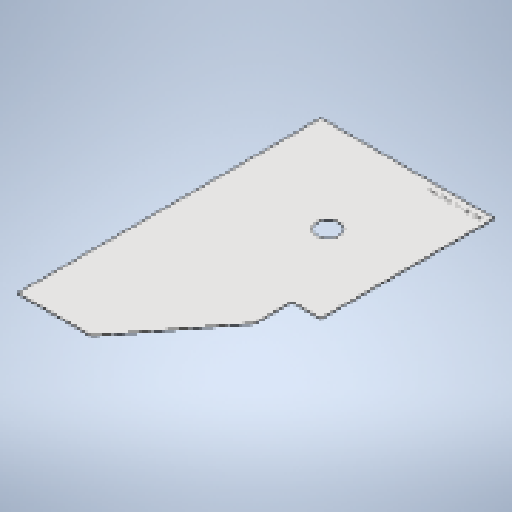
# Autodesk Inventor part: TRM 015 left board main
Saved by Autodesk Inventor 2025 (Build 290162010, 162A)
## iProperties
Created: 2024-08-07
Part Number: TRM 015 left board main
Material: AISI 304
Document SubType Name: Sheet Metal
Designer: pokla
Density: 8.02768 g/cm^3
Flat Pattern Width: 60.129 cm
Flat Pattern Length: 105 cm
Flat Pattern Area: 6313.54 cm^2
Sheet Metal Rule: AISI304 2mm Die16
Sheet Metal Width: 601,290 mm
Sheet Metal Length: 1050,000 mm
Sheet Metal Area: 631354,486 mm^2
Appearance: Default
Stock Number: ТРМ 015 левый борт основное
Author: pokla
Autodesk Inventor part; units mm, degrees
ref_plane "YZ Plane" through (0, 0, 0) normal (1, 0, 0) x (0, 1, 0)
ref_plane "XZ Plane" through (0, 0, 0) normal (0, 1, 0) x (-1, 0, 0)
ref_plane "XY Plane" through (0, 0, 0) normal (0, 0, 1) x (1, 0, 0)
sketch "Sketch1" plane through (0, 0, 0) normal (0, 0, 1) x (1, 0, 0)
  line L0 (-344.9768, -443.1916) -> (256.3132, -443.1916)
  line L1 (256.3132, -443.1916) -> (256.3132, 606.8084)
  line L2 (256.3132, 606.8084) -> (-344.9768, 606.8084)
  line L3 (-344.9768, 606.8084) -> (-344.9768, -443.1916)
  line L4 (-90.4868, -443.1916) -> (256.3132, 5.4517)
  circle A0 centre (0, 286.8084) radius 40
  line L5 (256.3132, 5.4517) -> (156.3132, 5.4517)
  line L6 (156.3132, 5.4517) -> (156.3132, -123.9149)
  point P0 (0, 0)
  dimension "d1" = 1050
  dimension "d14" = 80
  dimension "d15" = 320
  dimension "d16" = 100
  measures "d1" distance of L1.end L0.end
  measures "d14" diameter of A0
  measures "d15" distance from line of A0.centre L2
  measures "d16" distance of L4.end L5.end
extrude "Plate1" add sketch "Sketch1" along normal blind 2 contours L3 L2 L1 L5 L6 L4 L0
sketch "Sketch2" plane through (0, 0, 0) normal (0, 0, -1) x (-1, 0, 0)
  line L0 (-236.3132, 586.8084) -> (-36.3132, 586.8084) construction
  line L1 (-36.3132, 586.8084) -> (-36.3132, 566.8084) construction
  line L2 (-36.3132, 566.8084) -> (-236.3132, 566.8084) construction
  line L3 (-236.3132, 566.8084) -> (-236.3132, 586.8084) construction
  line L4 (-256.3132, 606.8084) -> (344.9768, 606.8084) projected
  line L5 (-256.3132, 5.4517) -> (-256.3132, 606.8084) projected
  point P0 (0, 0)
  point P1 (-48, 100)
  point P2 (-251, -525)
  point P3 (-50, 98)
  dimension "d6" = 200
  dimension "d9" = 20
  dimension "d10" = 20
  dimension "d11" = 20
  constraints: 4 other
  measures "d6" distance of L0.start L0.end
  measures "d9" distance of L0.end L1.end
  measures "d11" length of L3
mark "Mark1"
equation "\"d2\" = Thickness"
equation "\"BendReliefWidth\" = Thickness"
equation "\"BendReliefDepth\" = 0.5 * Thickness"
equation "\"CornerReliefSize\" = 4 * Thickness"
equation "\"MinimumRemnant\" = 2 * Thickness"
equation "\"TransitionRadius\" = BendRadius"
equation "\"JacobiRadiusSize\" = BendRadius"
equation "\"GapSize\" = Thickness"
equation "\"Thickness\" = 2"
equation "\"BendRadius\" = 2.75"
body "Solid1"
